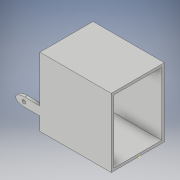
# Autodesk Inventor part: Tape measure holder case Albert
Saved by Autodesk Inventor 2019 (Build 230136000, 136)
## iProperties
Created: 2018-11-07
Part Number: Tape measure holder case Albert
Material: Generic
Document SubType Name: Modeling
Designer: mrhftc
Density: 1 g/cm^3
Appearance: Default
Author: mrhftc
Autodesk Inventor part; units mm, degrees
ref_plane "YZ Plane" through (0, 0, 0) normal (1, 0, 0) x (0, 1, 0)
ref_plane "XZ Plane" through (0, 0, 0) normal (0, 1, 0) x (-1, 0, 0)
ref_plane "XY Plane" through (0, 0, 0) normal (0, 0, 1) x (1, 0, 0)
sketch "Sketch1" plane through (0, 0, 0) normal (0, 1, 0) x (-1, 0, 0)
  line L0 (11.9219, 31.3255) -> (-68.5781, 31.3255)
  line L1 (-68.5781, 31.3255) -> (-68.5781, -28.6745)
  line L2 (-68.5781, -28.6745) -> (11.9219, -28.6745)
  line L3 (11.9219, -28.6745) -> (11.9219, 31.3255)
  point P0 (0, 0)
  dimension "d0" = 60
  dimension "d1" = 80.5
  constraints: 8 end point, 2 parallel, 1 horizontal, 1 perpendicular
  measures "d0" distance of L2.end L0.start
  measures "d1" distance of L0.start L0.end
extrude "Extrusion1" add sketch "Sketch1" along normal blind 77.4
sketch "Sketch2" plane through (68.5781, 0, 31.3255) normal (1, 0, 0) x (0, 0, -1)
  line L0 (3, 74.4) -> (57, 74.4)
  line L1 (57, 74.4) -> (57, 3)
  line L2 (57, 3) -> (3, 3)
  line L3 (3, 3) -> (3, 74.4)
  line L4 (0, 77.4) -> (60, 77.4) projected
  line L5 (0, 0) -> (0, 77.4) projected
  point P0 (31.3255, 0)
  dimension "d4" = 54
  dimension "d5" = 71.4
  dimension "d6" = 3
  dimension "d7" = 3
  constraints: 8 end point, 2 parallel, 1 horizontal, 1 perpendicular
  measures "d4" distance of L0.start L0.end
  measures "d5" distance of L0.end L1.end
  measures "d6" distance between parallel lines of L4 L0
  measures "d7" distance between parallel lines of L5 L3
sketch "Sketch3" plane through (68.5781, 0, 31.3255) normal (1, 0, 0) x (0, 0, -1)
  point P0 (31.3255, 0)
extrude "Extrusion2" cut sketch "Sketch2" against normal blind 74.5
sketch "Sketch4" plane through (-11.9219, 0, 31.3255) normal (0, 0, 1) x (1, 0, 0)
  line L0 (0, 15) -> (-17, 15)
  line L1 (-17, 15) -> (-17, 25)
  line L2 (-17, 25) -> (0, 25)
  line L3 (0, 25) -> (0, 15)
  ellipse E0 centre (-17, 20) end of major axis (-17, 15) minor radius 10.4512
  line L4 (0, 0) -> (0, 77.4) projected
  line L5 (0, 0) -> (80.5, 0) projected
  point P0 (11.9219, 0)
  dimension "d10" = 17
  dimension "d11" = 10
  dimension "d12" = 0
  dimension "d15" = 15
  constraints: 8 end point, 2 parallel, 1 horizontal, 1 midpoint, 1 perpendicular, 1 vertical, 1 vertical alignment, 2 other
  measures "d10" distance of L1.end L2.end
  measures "d11" distance of L2.end L0.start
  measures "d12" distance between parallel lines of L4 L3
  measures "d15" distance between parallel lines of L5 L0
extrude "Extrusion3" add sketch "Sketch4" against normal blind 3
sketch "Sketch7" plane through (-11.9219, 0, 31.3255) normal (0, 0, 1) x (1, 0, 0)
  circle A0 centre (-18.0318, 20) radius 2
  line L0 (0, 15) -> (-17, 15) projected
  point P0 (11.9219, 0)
  dimension "d16" = 4
  dimension "d17" = 5
  constraints: 1 centre point
  measures "d16" diameter of A0
  measures "d17" distance from line of L0 A0.centre
extrude "Extrusion4" cut sketch "Sketch7" against normal blind 3
body "Solid1"
